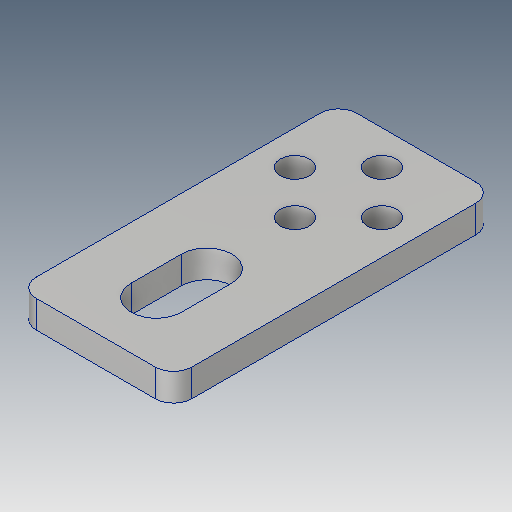
# Autodesk Inventor part: LimitSwitchMount
Saved by Autodesk Inventor 2020.3 (Build 243373000, 373)
## iProperties
Created: 2021-10-04
Part Number: LimitSwitchMount
Material: Aluminum 6061
Document SubType Name: Sheet Metal
Designer: justi
Density: 2.7 g/cm^3
Sheet Metal Rule: Default_mm
Appearance: Aluminum - Flat
Mass: 4.09364 g
Surface Area: 15.1795 cm^2
Volume: 1.51616 cm^3
Author: justi
Autodesk Inventor part; units mm, degrees
ref_plane "YZ Plane" through (0, 0, 0) normal (1, 0, 0) x (0, 1, 0)
ref_plane "XZ Plane" through (0, 0, 0) normal (0, 1, 0) x (-1, 0, 0)
sketch "Sketch1" plane through (0, 0, 0) normal (0, 1, 0) x (-1, 0, 0)
  line L0 (8.5, 17.5) -> (-8.5, 17.5)
  line L1 (-8.5, 17.5) -> (-8.5, -17.5)
  line L2 (-8.5, -17.5) -> (8.5, -17.5)
  line L3 (8.5, -17.5) -> (8.5, 17.5)
  line L4 (8.5, 17.5) -> (-8.5, -17.5) construction
  line L5 (-8.5, 17.5) -> (8.5, -17.5) construction
  line L6 (0, -17.5) -> (0, -0.5)
  line L7 (0, -9) -> (4.75, -9) construction
  circle A0 centre (0, -9) radius 4.75 construction
  line L8 (0, 10.8819) -> (0, 5.3819) construction
  line L9 (-2.75, 10.8819) -> (-2.75, 5.3819)
  line L10 (2.75, 5.3819) -> (2.75, 10.8819)
  arc A1 (2.75, 10.8819) -> (-2.75, 10.8819) centre (0, 10.8819) ccw
  arc A2 (-2.75, 5.3819) -> (2.75, 5.3819) centre (0, 5.3819) ccw
  point P0 (0, 0)
  point P1 (0, -4.25)
  point P2 (0, -13.75)
  point P3 (-4.75, -9)
  point P4 (0, 8.1319)
  dimension "d0" = 17
  dimension "d1" = 35
  dimension "d2" = 17
  dimension "d3" = 4.75
  dimension "d4" = 2.75
  dimension "d5" = 5.5
  constraints: 24 end point, 8 point on circle, 5 midpoint, 4 tangent, 3 centre point, 3 parallel, 2 coincident, 2 horizontal, 2 point on line, 2 vertical, 1 perpendicular
  measures "d0" distance of L2.end L1.end
  measures "d1" distance of L1.end L0.end
  measures "d2" distance of L6.start L6.end
  measures "d3" distance of L7.start L7.end
  measures "d4" distance of point (0, 8.132) L8.end
  measures "d5" diameter of A2
extrude "Plate1" add sketch "Sketch1" along normal blind 3
hole "Hole1" at (0, 0, -4.25) at (0, 0, -13.75) at (-4.75, 0, -9) at (4.75, 0, -9) direction (0, 1, 0) diameter 3.2 depth 3 tip angle 118
fillet "Fillet1" radius 2 4 edges at (-8.5, 1.5, 17.5) (8.5, 1.5, 17.5) (-8.5, 1.5, -17.5) (8.5, 1.5, -17.5)
ref_plane "Work Plane1" through (0, 0, 5.3819) normal (-1, 0, 0) x (0, 0, 1)
equation "\"d12\" = Thickness"
equation "\"d6\" = Thickness"
equation "\"BendRadius\" = Thickness"
equation "\"BendReliefWidth\" = Thickness"
equation "\"BendReliefDepth\" = 0.5 * Thickness"
equation "\"CornerReliefSize\" = 4 * Thickness"
equation "\"MinimumRemnant\" = 2 * Thickness"
equation "\"TransitionRadius\" = BendRadius"
equation "\"JacobiRadiusSize\" = BendRadius"
equation "\"GapSize\" = Thickness"
equation "\"Thickness\" = 3"
body "Solid1"
